Autodesk Fusion 360 part; units mm, degrees
(part 5 of 7)
  line L387 (58.5414, -43.6372) -> (58.5794, -43.7007)
  line L388 (58.5794, -43.7007) -> (58.6195, -43.7622)
  line L389 (58.6195, -43.7622) -> (58.6622, -43.8212)
  line L390 (58.6622, -43.8212) -> (58.7086, -43.8765)
  line L391 (58.7086, -43.8765) -> (59.0247, -44.1929)
  line L392 (59.0247, -44.1929) -> (58.8773, -44.3441)
  line L393 (58.8773, -44.3441) -> (58.734, -44.4991)
  line L394 (58.734, -44.4991) -> (58.5948, -44.6578)
  line L395 (58.5948, -44.6578) -> (58.4598, -44.8202)
  line L396 (58.4598, -44.8202) -> (58.1122, -44.5389)
  line L397 (58.1122, -44.5389) -> (58.0523, -44.4985)
  line L398 (58.0523, -44.4985) -> (57.9892, -44.4623)
  line L399 (57.9892, -44.4623) -> (57.9238, -44.4288)
  line L400 (57.9238, -44.4288) -> (57.8567, -44.3976)
  line L401 (57.8567, -44.3976) -> (57.788, -44.3685)
  line L402 (57.788, -44.3685) -> (57.7178, -44.3412)
  line L403 (57.7178, -44.3412) -> (57.6464, -44.3157)
  line L404 (57.6464, -44.3157) -> (57.5738, -44.2918)
  line L405 (57.5738, -44.2918) -> (57.5, -44.2695)
  line L406 (57.5, -44.2695) -> (57.4251, -44.2487)
  line L407 (57.4251, -44.2487) -> (57.3492, -44.2295)
  line L408 (57.3492, -44.2295) -> (57.2723, -44.2117)
  line L409 (57.2723, -44.2117) -> (57.188, -44.324)
  line L410 (57.188, -44.324) -> (57.1055, -44.4376)
  line L411 (57.1055, -44.4376) -> (57.0247, -44.5525)
  line L412 (57.0247, -44.5525) -> (57.0654, -44.6201)
  line L413 (57.0654, -44.6201) -> (57.1071, -44.6863)
  line L414 (57.1071, -44.6863) -> (57.15, -44.7511)
  line L415 (57.15, -44.7511) -> (57.194, -44.8144)
  line L416 (57.194, -44.8144) -> (57.2392, -44.8762)
  line L417 (57.2392, -44.8762) -> (57.2856, -44.9362)
  line L418 (57.2856, -44.9362) -> (57.3332, -44.9945)
  line L419 (57.3332, -44.9945) -> (57.3821, -45.0508)
  line L420 (57.3821, -45.0508) -> (57.4325, -45.105)
  line L421 (57.4325, -45.105) -> (57.4846, -45.1568)
  line L422 (57.4846, -45.1568) -> (57.5385, -45.2057)
  line L423 (57.5385, -45.2057) -> (57.5954, -45.2502)
  line L424 (57.5954, -45.2502) -> (57.9704, -45.4939)
  line L425 (57.9704, -45.4939) -> (57.8577, -45.6724)
  line L426 (57.8577, -45.6724) -> (57.7497, -45.8538)
  line L427 (57.7497, -45.8538) -> (57.6466, -46.038)
  line L428 (57.6466, -46.038) -> (57.5483, -46.2249)
  line L429 (57.5483, -46.2249) -> (57.1498, -46.022)
  line L430 (57.1498, -46.022) -> (57.0828, -45.995)
  line L431 (57.0828, -45.995) -> (57.0135, -45.9727)
  line L432 (57.0135, -45.9727) -> (56.9427, -45.9535)
  line L433 (56.9427, -45.9535) -> (56.8705, -45.937)
  line L434 (56.8705, -45.937) -> (56.7972, -45.9228)
  line L435 (56.7972, -45.9228) -> (56.723, -45.9107)
  line L436 (56.723, -45.9107) -> (56.6478, -45.9005)
  line L437 (56.6478, -45.9005) -> (56.5717, -45.8923)
  line L438 (56.5717, -45.8923) -> (56.4949, -45.8858)
  line L439 (56.4949, -45.8858) -> (56.4174, -45.8811)
  line L440 (56.4174, -45.8811) -> (56.3391, -45.878)
  line L441 (56.3391, -45.878) -> (56.2602, -45.8766)
  line L442 (56.2602, -45.8766) -> (56.2011, -46.004)
  line L443 (56.2011, -46.004) -> (56.144, -46.1323)
  line L444 (56.144, -46.1323) -> (56.0888, -46.2614)
  line L445 (56.0888, -46.2614) -> (56.1427, -46.3191)
  line L446 (56.1427, -46.3191) -> (56.1973, -46.3752)
  line L447 (56.1973, -46.3752) -> (56.2528, -46.4297)
  line L448 (56.2528, -46.4297) -> (56.309, -46.4825)
  line L449 (56.309, -46.4825) -> (56.366, -46.5334)
  line L450 (56.366, -46.5334) -> (56.4238, -46.5825)
  line L451 (56.4238, -46.5825) -> (56.4825, -46.6296)
  line L452 (56.4825, -46.6296) -> (56.5421, -46.6746)
  line L453 (56.5421, -46.6746) -> (56.6027, -46.7171)
  line L454 (56.6027, -46.7171) -> (56.6644, -46.757)
  line L455 (56.6644, -46.757) -> (56.7273, -46.7936)
  line L456 (56.7273, -46.7936) -> (56.7922, -46.8252)
  line L457 (56.7922, -46.8252) -> (57.2096, -46.9856)
  line L458 (57.2096, -46.9856) -> (57.1365, -47.1837)
  line L459 (57.1365, -47.1837) -> (57.0686, -47.3836)
  line L460 (57.0686, -47.3836) -> (57.006, -47.5852)
  line L461 (57.006, -47.5852) -> (56.9488, -47.7885)
  line L462 (56.9488, -47.7885) -> (56.5167, -47.6729)
  line L463 (56.5167, -47.6729) -> (56.4457, -47.6603)
  line L464 (56.4457, -47.6603) -> (56.3732, -47.6529)
  line L465 (56.3732, -47.6529) -> (56.2999, -47.6489)
  line L466 (56.2999, -47.6489) -> (56.2259, -47.6478)
  line L467 (56.2259, -47.6478) -> (56.1513, -47.6491)
  line L468 (56.1513, -47.6491) -> (56.0761, -47.6527)
  line L469 (56.0761, -47.6527) -> (56.0005, -47.6584)
  line L470 (56.0005, -47.6584) -> (55.9244, -47.6661)
  line L471 (55.9244, -47.6661) -> (55.8479, -47.6758)
  line L472 (55.8479, -47.6758) -> (55.771, -47.6873)
  line L473 (55.771, -47.6873) -> (55.6939, -47.7005)
  line L474 (55.6939, -47.7005) -> (55.6164, -47.7156)
  line L475 (55.6164, -47.7156) -> (55.5851, -47.8525)
  line L476 (55.5851, -47.8525) -> (55.5559, -47.9898)
  line L477 (55.5559, -47.9898) -> (55.5288, -48.1276)
  line L478 (55.5288, -48.1276) -> (55.5935, -48.1728)
  line L479 (55.5935, -48.1728) -> (55.6586, -48.2164)
  line L480 (55.6586, -48.2164) -> (55.7241, -48.2581)
  line L481 (55.7241, -48.2581) -> (55.79, -48.2981)
  line L482 (55.79, -48.2981) -> (55.8564, -48.3361)
  line L483 (55.8564, -48.3361) -> (55.9232, -48.3721)
  line L484 (55.9232, -48.3721) -> (55.9904, -48.4059)
  line L485 (55.9904, -48.4059) -> (56.058, -48.4375)
  line L486 (56.058, -48.4375) -> (56.1261, -48.4665)
  line L487 (56.1261, -48.4665) -> (56.1947, -48.4927)
  line L488 (56.1947, -48.4927) -> (56.2639, -48.5154)
  line L489 (56.2639, -48.5154) -> (56.3339, -48.5328)
  line L490 (56.3339, -48.5328) -> (56.7757, -48.603)
  line L491 (56.7757, -48.603) -> (56.7453, -48.8119)
  line L492 (56.7453, -48.8119) -> (56.7205, -49.0216)
  line L493 (56.7205, -49.0216) -> (56.7012, -49.2318)
  line L494 (56.7012, -49.2318) -> (56.6874, -49.4425)
  line L495 (56.6874, -49.4425) -> (56.2408, -49.4192)
  line L496 (56.2408, -49.4192) -> (56.1687, -49.4218)
  line L497 (56.1687, -49.4218) -> (56.0963, -49.4296)
  line L498 (56.0963, -49.4296) -> (56.0237, -49.4409)
  line L499 (56.0237, -49.4409) -> (55.9511, -49.4551)
  line L500 (55.9511, -49.4551) -> (55.8784, -49.472)
  line L501 (55.8784, -49.472) -> (55.8056, -49.4911)
  line L502 (55.8056, -49.4911) -> (55.7328, -49.5124)
  line L503 (55.7328, -49.5124) -> (55.66, -49.5358)
  line L504 (55.66, -49.5358) -> (55.5871, -49.5611)
  line L505 (55.5871, -49.5611) -> (55.5144, -49.5884)
  line L506 (55.5144, -49.5884) -> (55.4416, -49.6174)
  line L507 (55.4416, -49.6174) -> (55.369, -49.6482)
  line L508 (55.369, -49.6482) -> (55.3669, -49.7886)
  line L509 (55.3669, -49.7886) -> (55.3669, -49.929)
  line L510 (55.3669, -49.929) -> (55.369, -50.0695)
  line L511 (55.369, -50.0695) -> (55.4416, -50.1003)
  line L512 (55.4416, -50.1003) -> (55.5144, -50.1293)
  line L513 (55.5144, -50.1293) -> (55.5871, -50.1565)
  line L514 (55.5871, -50.1565) -> (55.66, -50.1819)
  line L515 (55.66, -50.1819) -> (55.7328, -50.2052)
  line L516 (55.7328, -50.2052) -> (55.8056, -50.2266)
  line L517 (55.8056, -50.2266) -> (55.8784, -50.2457)
  line L518 (55.8784, -50.2457) -> (55.9511, -50.2625)
  line L519 (55.9511, -50.2625) -> (56.0237, -50.2768)
  line L520 (56.0237, -50.2768) -> (56.0963, -50.2881)
  line L521 (56.0963, -50.2881) -> (56.1687, -50.2959)
  line L522 (56.1687, -50.2959) -> (56.2408, -50.2984)
  line L523 (56.2408, -50.2984) -> (56.6874, -50.2752)
  line L524 (56.6874, -50.2752) -> (56.7012, -50.4859)
  line L525 (56.7012, -50.4859) -> (56.7205, -50.6961)
  line L526 (56.7205, -50.6961) -> (56.7453, -50.9058)
  line L527 (56.7453, -50.9058) -> (56.7757, -51.1147)
  line L528 (56.7757, -51.1147) -> (56.3339, -51.1848)
  line L529 (56.3339, -51.1848) -> (56.2639, -51.2023)
  line L530 (56.2639, -51.2023) -> (56.1947, -51.225)
  line L531 (56.1947, -51.225) -> (56.1261, -51.2511)
  line L532 (56.1261, -51.2511) -> (56.058, -51.2802)
  line L533 (56.058, -51.2802) -> (55.9904, -51.3117)
  line L534 (55.9904, -51.3117) -> (55.9232, -51.3456)
  line L535 (55.9232, -51.3456) -> (55.8564, -51.3816)
  line L536 (55.8564, -51.3816) -> (55.79, -51.4196)
  line L537 (55.79, -51.4196) -> (55.7241, -51.4595)
  line L538 (55.7241, -51.4595) -> (55.6586, -51.5013)
  line L539 (55.6586, -51.5013) -> (55.5935, -51.5448)
  line L540 (55.5935, -51.5448) -> (55.5288, -51.59)
  line L541 (55.5288, -51.59) -> (55.5559, -51.7278)
  line L542 (55.5559, -51.7278) -> (55.5851, -51.8652)
  line L543 (55.5851, -51.8652) -> (55.6164, -52.0021)
  line L544 (55.6164, -52.0021) -> (55.6939, -52.0171)
  line L545 (55.6939, -52.0171) -> (55.771, -52.0304)
  line L546 (55.771, -52.0304) -> (55.8479, -52.0419)
  line L547 (55.8479, -52.0419) -> (55.9244, -52.0515)
  line L548 (55.9244, -52.0515) -> (56.0005, -52.0593)
  line L549 (56.0005, -52.0593) -> (56.0761, -52.065)
  line L550 (56.0761, -52.065) -> (56.1513, -52.0686)
  line L551 (56.1513, -52.0686) -> (56.2259, -52.0699)
  line L552 (56.2259, -52.0699) -> (56.2999, -52.0687)
  line L553 (56.2999, -52.0687) -> (56.3732, -52.0647)
  line L554 (56.3732, -52.0647) -> (56.4457, -52.0573)
  line L555 (56.4457, -52.0573) -> (56.5167, -52.0448)
  line L556 (56.5167, -52.0448) -> (56.9488, -51.9292)
  line L557 (56.9488, -51.9292) -> (57.006, -52.1324)
  line L558 (57.006, -52.1324) -> (57.0686, -52.3341)
  line L559 (57.0686, -52.3341) -> (57.1365, -52.534)
  line L560 (57.1365, -52.534) -> (57.2096, -52.732)
  line L561 (57.2096, -52.732) -> (56.7922, -52.8925)
  line L562 (56.7922, -52.8925) -> (56.7273, -52.9241)
  line L563 (56.7273, -52.9241) -> (56.6644, -52.9607)
  line L564 (56.6644, -52.9607) -> (56.6027, -53.0005)
  line L565 (56.6027, -53.0005) -> (56.5421, -53.0431)
  line L566 (56.5421, -53.0431) -> (56.4825, -53.088)
  line L567 (56.4825, -53.088) -> (56.4238, -53.1351)
  line L568 (56.4238, -53.1351) -> (56.366, -53.1842)
  line L569 (56.366, -53.1842) -> (56.309, -53.2352)
  line L570 (56.309, -53.2352) -> (56.2528, -53.288)
  line L571 (56.2528, -53.288) -> (56.1973, -53.3424)
  line L572 (56.1973, -53.3424) -> (56.1427, -53.3985)
  line L573 (56.1427, -53.3985) -> (56.0888, -53.4562)
  line L574 (56.0888, -53.4562) -> (56.144, -53.5854)
  line L575 (56.144, -53.5854) -> (56.2011, -53.7137)
  line L576 (56.2011, -53.7137) -> (56.2602, -53.8411)
  line L577 (56.2602, -53.8411) -> (56.3391, -53.8396)
  line L578 (56.3391, -53.8396) -> (56.4174, -53.8366)
  line L579 (56.4174, -53.8366) -> (56.4949, -53.8319)
  line L580 (56.4949, -53.8319) -> (56.5717, -53.8254)
  line L581 (56.5717, -53.8254) -> (56.6478, -53.8171)
  line L582 (56.6478, -53.8171) -> (56.723, -53.807)
  line L583 (56.723, -53.807) -> (56.7972, -53.7949)
  line L584 (56.7972, -53.7949) -> (56.8705, -53.7807)
  line L585 (56.8705, -53.7807) -> (56.9427, -53.7641)
  line L586 (56.9427, -53.7641) -> (57.0135, -53.745)
  line L587 (57.0135, -53.745) -> (57.0828, -53.7227)
  line L588 (57.0828, -53.7227) -> (57.1498, -53.6956)
  line L589 (57.1498, -53.6956) -> (57.5483, -53.4927)
  line L590 (57.5483, -53.4927) -> (57.6466, -53.6796)
  line L591 (57.6466, -53.6796) -> (57.7497, -53.8638)
  line L592 (57.7497, -53.8638) -> (57.8577, -54.0453)
  line L593 (57.8577, -54.0453) -> (57.9704, -54.2238)
  line L594 (57.9704, -54.2238) -> (57.5954, -54.4675)
  line L595 (57.5954, -54.4675) -> (57.5385, -54.5119)
  line L596 (57.5385, -54.5119) -> (57.4846, -54.5608)
  line L597 (57.4846, -54.5608) -> (57.4325, -54.6126)
  line L598 (57.4325, -54.6126) -> (57.3821, -54.6668)
  line L599 (57.3821, -54.6668) -> (57.3332, -54.7232)
  line L600 (57.3332, -54.7232) -> (57.2856, -54.7815)
  line L601 (57.2856, -54.7815) -> (57.2392, -54.8415)
  line L602 (57.2392, -54.8415) -> (57.194, -54.9032)
  line L603 (57.194, -54.9032) -> (57.15, -54.9665)
  line L604 (57.15, -54.9665) -> (57.1071, -55.0313)
  line L605 (57.1071, -55.0313) -> (57.0654, -55.0976)
  line L606 (57.0654, -55.0976) -> (57.0247, -55.1652)
  line L607 (57.0247, -55.1652) -> (57.1055, -55.28)
  line L608 (57.1055, -55.28) -> (57.188, -55.3936)
  line L609 (57.188, -55.3936) -> (57.2723, -55.506)
  line L610 (57.2723, -55.506) -> (57.3492, -55.4882)
  line L611 (57.3492, -55.4882) -> (57.4251, -55.4689)
  line L612 (57.4251, -55.4689) -> (57.5, -55.4482)
  line L613 (57.5, -55.4482) -> (57.5738, -55.4259)
  line L614 (57.5738, -55.4259) -> (57.6464, -55.402)
  line L615 (57.6464, -55.402) -> (57.7178, -55.3765)
  line L616 (57.7178, -55.3765) -> (57.788, -55.3492)
  line L617 (57.788, -55.3492) -> (57.8567, -55.32)
  line L618 (57.8567, -55.32) -> (57.9238, -55.2888)
  line L619 (57.9238, -55.2888) -> (57.9892, -55.2554)
  line L620 (57.9892, -55.2554) -> (58.0523, -55.2191)
  line L621 (58.0523, -55.2191) -> (58.1122, -55.1788)
  line L622 (58.1122, -55.1788) -> (58.4598, -54.8975)
  line L623 (58.4598, -54.8975) -> (58.5948, -55.0598)
  line L624 (58.5948, -55.0598) -> (58.734, -55.2186)
  line L625 (58.734, -55.2186) -> (58.8773, -55.3736)
  line L626 (58.8773, -55.3736) -> (59.0247, -55.5248)
  line L627 (59.0247, -55.5248) -> (58.7086, -55.8411)
  line L628 (58.7086, -55.8411) -> (58.6622, -55.8964)
  line L629 (58.6622, -55.8964) -> (58.6195, -55.9554)
  line L630 (58.6195, -55.9554) -> (58.5794, -56.0169)
  line L631 (58.5794, -56.0169) -> (58.5414, -56.0805)
  line L632 (58.5414, -56.0805) -> (58.5052, -56.1457)
  line L633 (58.5052, -56.1457) -> (58.4708, -56.2126)
  line L634 (58.4708, -56.2126) -> (58.4379, -56.281)
  line L635 (58.4379, -56.281) -> (58.4065, -56.3508)
  line L636 (58.4065, -56.3508) -> (58.3767, -56.4218)
  line L637 (58.3767, -56.4218) -> (58.3482, -56.4941)
  line L638 (58.3482, -56.4941) -> (58.3211, -56.5676)
  line L639 (58.3211, -56.5676) -> (58.2954, -56.6422)
  line L640 (58.2954, -56.6422) -> (58.3983, -56.7378)
  line L641 (58.3983, -56.7378) -> (58.5026, -56.8317)
  line L642 (58.5026, -56.8317) -> (58.6084, -56.9241)
  line L643 (58.6084, -56.9241) -> (58.6799, -56.8907)
  line L644 (58.6799, -56.8907) -> (58.7502, -56.8561)
  line L645 (58.7502, -56.8561) -> (58.8191, -56.8202)
  line L646 (58.8191, -56.8202) -> (58.8866, -56.7831)
  line L647 (58.8866, -56.7831) -> (58.9527, -56.7446)
  line L648 (58.9527, -56.7446) -> (59.0173, -56.7048)
  line L649 (59.0173, -56.7048) -> (59.0802, -56.6635)
  line L650 (59.0802, -56.6635) -> (59.1414, -56.6207)
  line L651 (59.1414, -56.6207) -> (59.2006, -56.5762)
  line L652 (59.2006, -56.5762) -> (59.2575, -56.5299)
  line L653 (59.2575, -56.5299) -> (59.3118, -56.4813)
  line L654 (59.3118, -56.4813) -> (59.3619, -56.4294)
  line L655 (59.3619, -56.4294) -> (59.6435, -56.082)
  line L656 (59.6435, -56.082) -> (59.8093, -56.2127)
  line L657 (59.8093, -56.2127) -> (59.9784, -56.3391)
  line L658 (59.9784, -56.3391) -> (60.1509, -56.4609)
  line L659 (60.1509, -56.4609) -> (60.3264, -56.5781)
  line L660 (60.3264, -56.5781) -> (60.083, -56.9533)
  line L661 (60.083, -56.9533) -> (60.0491, -57.017)
  line L662 (60.0491, -57.017) -> (60.0197, -57.0836)
  line L663 (60.0197, -57.0836) -> (59.9932, -57.1521)
  line L664 (59.9932, -57.1521) -> (59.9692, -57.2222)
  line L665 (59.9692, -57.2222) -> (59.9474, -57.2935)
  line L666 (59.9474, -57.2935) -> (59.9276, -57.3661)
  line L667 (59.9276, -57.3661) -> (59.9097, -57.4399)
  line L668 (59.9097, -57.4399) -> (59.8935, -57.5146)
  line L669 (59.8935, -57.5146) -> (59.8791, -57.5903)
  line L670 (59.8791, -57.5903) -> (59.8663, -57.667)
  line L671 (59.8663, -57.667) -> (59.855, -57.7445)
  line L672 (59.855, -57.7445) -> (59.8454, -57.8228)
  line L673 (59.8454, -57.8228) -> (59.9659, -57.8949)
  line L674 (59.9659, -57.8949) -> (60.0875, -57.9651)
  line L675 (60.0875, -57.9651) -> (60.2102, -58.0334)
  line L676 (60.2102, -58.0334) -> (60.2732, -57.9859)
  line L677 (60.2732, -57.9859) -> (60.3347, -57.9374)
  line L678 (60.3347, -57.9374) -> (60.3947, -57.888)
  line L679 (60.3947, -57.888) -> (60.453, -57.8376)
  line L680 (60.453, -57.8376) -> (60.5097, -57.7863)
  line L681 (60.5097, -57.7863) -> (60.5645, -57.7339)
  line L682 (60.5645, -57.7339) -> (60.6175, -57.6804)
  line L683 (60.6175, -57.6804) -> (60.6684, -57.6258)
  line L684 (60.6684, -57.6258) -> (60.7171, -57.57)
  line L685 (60.7171, -57.57) -> (60.7632, -57.5129)
  line L686 (60.7632, -57.5129) -> (60.8061, -57.4541)
  line L687 (60.8061, -57.4541) -> (60.8444, -57.3929)
  line L688 (60.8444, -57.3929) -> (61.0476, -56.9945)
  line L689 (61.0476, -56.9945) -> (61.2369, -57.0879)
  line L690 (61.2369, -57.0879) -> (61.4286, -57.1763)
  line L691 (61.4286, -57.1763) -> (61.6226, -57.2597)
  line L692 (61.6226, -57.2597) -> (61.8187, -57.3378)
  line L693 (61.8187, -57.3378) -> (61.6586, -57.7554)
  line L694 (61.6586, -57.7554) -> (61.6387, -57.8248)
  line L695 (61.6387, -57.8248) -> (61.6238, -57.8961)
  line L696 (61.6238, -57.8961) -> (61.6121, -57.9685)
  line L697 (61.6121, -57.9685) -> (61.6032, -58.042)
  line L698 (61.6032, -58.042) -> (61.5968, -58.1164)
  line L699 (61.5968, -58.1164) -> (61.5925, -58.1915)
  line L700 (61.5925, -58.1915) -> (61.5903, -58.2674)
  line L701 (61.5903, -58.2674) -> (61.59, -58.3438)
  line L702 (61.59, -58.3438) -> (61.5916, -58.4209)
  line L703 (61.5916, -58.4209) -> (61.595, -58.4986)
  line L704 (61.595, -58.4986) -> (61.6001, -58.5767)
  line L705 (61.6001, -58.5767) -> (61.607, -58.6553)
  line L706 (61.607, -58.6553) -> (61.7399, -58.7007)
  line L707 (61.7399, -58.7007) -> (61.8734, -58.7441)
  line L708 (61.8734, -58.7441) -> (62.0076, -58.7855)
  line L709 (62.0076, -58.7855) -> (62.0593, -58.7259)
  line L710 (62.0593, -58.7259) -> (62.1094, -58.6657)
  line L711 (62.1094, -58.6657) -> (62.1578, -58.6049)
  line L712 (62.1578, -58.6049) -> (62.2044, -58.5435)
  line L713 (62.2044, -58.5435) -> (62.2492, -58.4815)
  line L714 (62.2492, -58.4815) -> (62.2919, -58.4188)
  line L715 (62.2919, -58.4188) -> (62.3326, -58.3555)
  line L716 (62.3326, -58.3555) -> (62.3711, -58.2915)
  line L717 (62.3711, -58.2915) -> (62.4071, -58.2268)
  line L718 (62.4071, -58.2268) -> (62.4403, -58.1613)
  line L719 (62.4403, -58.1613) -> (62.4701, -58.0949)
  line L720 (62.4701, -58.0949) -> (62.4948, -58.0271)
  line L721 (62.4948, -58.0271) -> (62.6107, -57.5952)
  line L722 (62.6107, -57.5952) -> (62.8153, -57.6472)
  line L723 (62.8153, -57.6472) -> (63.0212, -57.6938)
  line L724 (63.0212, -57.6938) -> (63.2283, -57.735)
  line L725 (63.2283, -57.735) -> (63.4364, -57.7707)
  line L726 (63.4364, -57.7707) -> (63.3666, -58.2124)
  line L727 (63.3666, -58.2124) -> (63.3615, -58.2844)
  line L728 (63.3615, -58.2844) -> (63.3617, -58.3572)
  line L729 (63.3617, -58.3572) -> (63.3654, -58.4305)
  line L730 (63.3654, -58.4305) -> (63.372, -58.5043)
  line L731 (63.372, -58.5043) -> (63.3811, -58.5784)
  line L732 (63.3811, -58.5784) -> (63.3926, -58.6527)
  line L733 (63.3926, -58.6527) -> (63.4062, -58.7274)
  line L734 (63.4062, -58.7274) -> (63.4218, -58.8022)
  line L735 (63.4218, -58.8022) -> (63.4394, -58.8773)
  line L736 (63.4394, -58.8773) -> (63.4588, -58.9525)
  line L737 (63.4588, -58.9525) -> (63.4801, -59.0279)
  line L738 (63.4801, -59.0279) -> (63.5032, -59.1034)
  line L739 (63.5032, -59.1034) -> (63.6426, -59.1202)
  line L740 (63.6426, -59.1202) -> (63.7822, -59.1349)
  line L741 (63.7822, -59.1349) -> (63.9221, -59.1474)
  line L742 (63.9221, -59.1474) -> (63.9603, -59.0784)
  line L743 (63.9603, -59.0784) -> (63.9968, -59.0091)
  line L744 (63.9968, -59.0091) -> (64.0315, -58.9395)
  line L745 (64.0315, -58.9395) -> (64.0643, -58.8698)
  line L746 (64.0643, -58.8698) -> (64.0952, -58.7998)
  line L747 (64.0952, -58.7998) -> (64.124, -58.7296)
  line L748 (64.124, -58.7296) -> (64.1506, -58.6592)
  line L749 (64.1506, -58.6592) -> (64.175, -58.5887)
  line L750 (64.175, -58.5887) -> (64.1967, -58.5179)
  line L751 (64.1967, -58.5179) -> (64.2156, -58.447)
  line L752 (64.2156, -58.447) -> (64.2309, -58.3758)
  line L753 (64.2309, -58.3758) -> (64.241, -58.3043)
  line L754 (64.241, -58.3043) -> (64.2645, -57.8577)
  line L755 (64.2645, -57.8577) -> (64.4755, -57.866)
  line L756 (64.4755, -57.866) -> (64.6866, -57.8688)
  line L757 (64.6866, -57.8688) -> (64.8977, -57.866)
  line L758 (64.8977, -57.866) -> (65.1087, -57.8577)
  line L759 (65.1087, -57.8577) -> (65.1322, -58.3043)
  line L760 (65.1322, -58.3043) -> (65.1423, -58.3758)
  line L761 (65.1423, -58.3758) -> (65.1576, -58.447)
  line L762 (65.1576, -58.447) -> (65.1765, -58.5179)
  line L763 (65.1765, -58.5179) -> (65.1982, -58.5887)
  line L764 (65.1982, -58.5887) -> (65.2225, -58.6592)
  line L765 (65.2225, -58.6592) -> (65.2492, -58.7296)
  line L766 (65.2492, -58.7296) -> (65.278, -58.7998)
  line L767 (65.278, -58.7998) -> (65.3089, -58.8698)
  line L768 (65.3089, -58.8698) -> (65.3417, -58.9395)
  line L769 (65.3417, -58.9395) -> (65.3764, -59.0091)
  line L770 (65.3764, -59.0091) -> (65.4128, -59.0784)
  line L771 (65.4128, -59.0784) -> (65.4511, -59.1474)
  line L772 (65.4511, -59.1474) -> (65.5909, -59.1349)
  line L773 (65.5909, -59.1349) -> (65.7306, -59.1202)
  line L774 (65.7306, -59.1202) -> (65.87, -59.1034)
  line L775 (65.87, -59.1034) -> (65.8931, -59.0279)
  line L776 (65.8931, -59.0279) -> (65.9143, -58.9525)
  line L777 (65.9143, -58.9525) -> (65.9338, -58.8773)
  line L778 (65.9338, -58.8773) -> (65.9514, -58.8022)
  line L779 (65.9514, -58.8022) -> (65.967, -58.7274)
  line L780 (65.967, -58.7274) -> (65.9806, -58.6527)
  line L781 (65.9806, -58.6527) -> (65.9921, -58.5784)
  line L782 (65.9921, -58.5784) -> (66.0012, -58.5043)
  line L783 (66.0012, -58.5043) -> (66.0077, -58.4305)
  line L784 (66.0077, -58.4305) -> (66.0114, -58.3572)
  line L785 (66.0114, -58.3572) -> (66.0116, -58.2844)
  line L786 (66.0116, -58.2844) -> (66.0066, -58.2124)
  line L787 (66.0066, -58.2124) -> (65.9368, -57.7707)
  line L788 (65.9368, -57.7707) -> (66.1449, -57.735)
  line L789 (66.1449, -57.735) -> (66.352, -57.6938)
  line L790 (66.352, -57.6938) -> (66.5579, -57.6472)
  line L791 (66.5579, -57.6472) -> (66.7625, -57.5952)
  line L792 (66.7625, -57.5952) -> (66.8784, -58.0271)
  line L793 (66.8784, -58.0271) -> (66.9031, -58.0949)
  line L794 (66.9031, -58.0949) -> (66.9329, -58.1613)
  line L795 (66.9329, -58.1613) -> (66.9661, -58.2268)
  line L796 (66.9661, -58.2268) -> (67.0021, -58.2915)
  line L797 (67.0021, -58.2915) -> (67.0405, -58.3555)
  line L798 (67.0405, -58.3555) -> (67.0812, -58.4188)
  line L799 (67.0812, -58.4188) -> (67.124, -58.4815)
  line L800 (67.124, -58.4815) -> (67.1688, -58.5435)
  line L801 (67.1688, -58.5435) -> (67.2154, -58.6049)
  line L802 (67.2154, -58.6049) -> (67.2637, -58.6657)
  line L803 (67.2637, -58.6657) -> (67.3138, -58.7259)
  line L804 (67.3138, -58.7259) -> (67.3656, -58.7855)
  line L805 (67.3656, -58.7855) -> (67.4998, -58.7441)
  line L806 (67.4998, -58.7441) -> (67.6333, -58.7007)
  line L807 (67.6333, -58.7007) -> (67.7662, -58.6553)
  line L808 (67.7662, -58.6553) -> (67.773, -58.5767)
  line L809 (67.773, -58.5767) -> (67.7782, -58.4986)
  line L810 (67.7782, -58.4986) -> (67.7816, -58.4209)
  line L811 (67.7816, -58.4209) -> (67.7832, -58.3438)
  line L812 (67.7832, -58.3438) -> (67.7829, -58.2674)
  line L813 (67.7829, -58.2674) -> (67.7807, -58.1915)
  line L814 (67.7807, -58.1915) -> (67.7764, -58.1164)
  line L815 (67.7764, -58.1164) -> (67.7699, -58.042)
  line L816 (67.7699, -58.042) -> (67.761, -57.9685)
  line L817 (67.761, -57.9685) -> (67.7494, -57.8961)
  line L818 (67.7494, -57.8961) -> (67.7344, -57.8248)
  line L819 (67.7344, -57.8248) -> (67.7146, -57.7554)
  line L820 (67.7146, -57.7554) -> (67.5544, -57.3378)
  line L821 (67.5544, -57.3378) -> (67.7506, -57.2597)
  line L822 (67.7506, -57.2597) -> (67.9445, -57.1763)
  line L823 (67.9445, -57.1763) -> (68.1363, -57.0879)
  line L824 (68.1363, -57.0879) -> (68.3256, -56.9945)
  line L825 (68.3256, -56.9945) -> (68.5288, -57.3929)
  line L826 (68.5288, -57.3929) -> (68.567, -57.4541)
  line L827 (68.567, -57.4541) -> (68.61, -57.5129)
  line L828 (68.61, -57.5129) -> (68.6561, -57.57)
  line L829 (68.6561, -57.57) -> (68.7047, -57.6258)
  line L830 (68.7047, -57.6258) -> (68.7557, -57.6804)
  line L831 (68.7557, -57.6804) -> (68.8086, -57.7339)
  line L832 (68.8086, -57.7339) -> (68.8635, -57.7863)
  line L833 (68.8635, -57.7863) -> (68.9202, -57.8376)
  line L834 (68.9202, -57.8376) -> (68.9785, -57.888)
  line L835 (68.9785, -57.888) -> (69.0385, -57.9374)
  line L836 (69.0385, -57.9374) -> (69.1, -57.9859)
  line L837 (69.1, -57.9859) -> (69.163, -58.0334)
  line L838 (69.163, -58.0334) -> (69.2856, -57.9651)
  line L839 (69.2856, -57.9651) -> (69.4073, -57.8949)
  line L840 (69.4073, -57.8949) -> (69.5278, -57.8228)
  line L841 (69.5278, -57.8228) -> (69.5181, -57.7445)
  line L842 (69.5181, -57.7445) -> (69.5069, -57.667)
  line L843 (69.5069, -57.667) -> (69.4941, -57.5903)
  line L844 (69.4941, -57.5903) -> (69.4796, -57.5146)
  line L845 (69.4796, -57.5146) -> (69.4635, -57.4399)
  line L846 (69.4635, -57.4399) -> (69.4456, -57.3661)
  line L847 (69.4456, -57.3661) -> (69.4257, -57.2935)
  line L848 (69.4257, -57.2935) -> (69.4039, -57.2222)
  line L849 (69.4039, -57.2222) -> (69.3799, -57.1521)
  line L850 (69.3799, -57.1521) -> (69.3535, -57.0836)
  line L851 (69.3535, -57.0836) -> (69.3241, -57.017)
  line L852 (69.3241, -57.017) -> (69.2902, -56.9533)
  line L853 (69.2902, -56.9533) -> (69.0467, -56.5781)
  line L854 (69.0467, -56.5781) -> (69.2223, -56.4609)
  line L855 (69.2223, -56.4609) -> (69.3947, -56.3391)
  line L856 (69.3947, -56.3391) -> (69.5639, -56.2127)
  line L857 (69.5639, -56.2127) -> (69.7297, -56.082)
  line L858 (69.7297, -56.082) -> (70.0112, -56.4294)
  line L859 (70.0112, -56.4294) -> (70.0614, -56.4813)
  line L860 (70.0614, -56.4813) -> (70.1156, -56.5299)
  line L861 (70.1156, -56.5299) -> (70.1726, -56.5762)
  line L862 (70.1726, -56.5762) -> (70.2318, -56.6207)
  line L863 (70.2318, -56.6207) -> (70.2929, -56.6635)
  line L864 (70.2929, -56.6635) -> (70.3559, -56.7048)
  line L865 (70.3559, -56.7048) -> (70.4204, -56.7446)
  line L866 (70.4204, -56.7446) -> (70.4865, -56.7831)
  line L867 (70.4865, -56.7831) -> (70.5541, -56.8202)
  line L868 (70.5541, -56.8202) -> (70.623, -56.8561)
  line L869 (70.623, -56.8561) -> (70.6933, -56.8907)
  line L870 (70.6933, -56.8907) -> (70.7648, -56.9241)
  line L871 (70.7648, -56.9241) -> (70.8705, -56.8317)
  line L872 (70.8705, -56.8317) -> (70.9749, -56.7378)
  line L873 (70.9749, -56.7378) -> (71.0778, -56.6422)
  line L874 (71.0778, -56.6422) -> (71.0521, -56.5676)
  line L875 (71.0521, -56.5676) -> (71.025, -56.4941)
  line L876 (71.025, -56.4941) -> (70.9965, -56.4218)
  line L877 (70.9965, -56.4218) -> (70.9666, -56.3508)
  line L878 (70.9666, -56.3508) -> (70.9353, -56.281)
  line L879 (70.9353, -56.281) -> (70.9024, -56.2126)
  line L880 (70.9024, -56.2126) -> (70.8679, -56.1457)
  line L881 (70.8679, -56.1457) -> (70.8318, -56.0805)
  line L882 (70.8318, -56.0805) -> (70.7937, -56.0169)
  line L883 (70.7937, -56.0169) -> (70.7536, -55.9554)
  line L884 (70.7536, -55.9554) -> (70.711, -55.8964)
  line L885 (70.711, -55.8964) -> (70.6646, -55.8411)
  line L886 (70.6646, -55.8411) -> (70.3485, -55.5248)
  line L887 (70.3485, -55.5248) -> (70.4959, -55.3736)
  line L888 (70.4959, -55.3736) -> (70.6392, -55.2186)
  line L889 (70.6392, -55.2186) -> (70.7784, -55.0598)
  line L890 (70.7784, -55.0598) -> (70.9133, -54.8975)
  line L891 (70.9133, -54.8975) -> (71.261, -55.1788)
  line L892 (71.261, -55.1788) -> (71.3208, -55.2191)
  line L893 (71.3208, -55.2191) -> (71.384, -55.2554)
  line L894 (71.384, -55.2554) -> (71.4493, -55.2888)
  line L895 (71.4493, -55.2888) -> (71.5165, -55.32)
  line L896 (71.5165, -55.32) -> (71.5852, -55.3492)
  line L897 (71.5852, -55.3492) -> (71.6553, -55.3765)
  line L898 (71.6553, -55.3765) -> (71.7268, -55.402)
  line L899 (71.7268, -55.402) -> (71.7994, -55.4259)
  line L900 (71.7994, -55.4259) -> (71.8732, -55.4482)
  line L901 (71.8732, -55.4482) -> (71.9481, -55.4689)
  line L902 (71.9481, -55.4689) -> (72.024, -55.4882)
  line L903 (72.024, -55.4882) -> (72.1009, -55.506)
  line L904 (72.1009, -55.506) -> (72.1851, -55.3936)
  line L905 (72.1851, -55.3936) -> (72.2677, -55.28)
  line L906 (72.2677, -55.28) -> (72.3485, -55.1652)
  line L907 (72.3485, -55.1652) -> (72.3078, -55.0976)
  line L908 (72.3078, -55.0976) -> (72.266, -55.0313)
  line L909 (72.266, -55.0313) -> (72.2232, -54.9665)
  line L910 (72.2232, -54.9665) -> (72.1792, -54.9032)
  line L911 (72.1792, -54.9032) -> (72.134, -54.8415)
  line L912 (72.134, -54.8415) -> (72.0876, -54.7815)
  line L913 (72.0876, -54.7815) -> (72.04, -54.7232)
  line L914 (72.04, -54.7232) -> (71.991, -54.6668)
  line L915 (71.991, -54.6668) -> (71.9406, -54.6126)
  line L916 (71.9406, -54.6126) -> (71.8886, -54.5608)
  line L917 (71.8886, -54.5608) -> (71.8346, -54.5119)
  line L918 (71.8346, -54.5119) -> (71.7778, -54.4675)
  line L919 (71.7778, -54.4675) -> (71.4028, -54.2238)
  line L920 (71.4028, -54.2238) -> (71.5155, -54.0453)
  line L921 (71.5155, -54.0453) -> (71.6234, -53.8638)
  line L922 (71.6234, -53.8638) -> (71.7266, -53.6796)
  line L923 (71.7266, -53.6796) -> (71.8248, -53.4927)
  line L924 (71.8248, -53.4927) -> (72.2234, -53.6956)
  line L925 (72.2234, -53.6956) -> (72.2903, -53.7227)
  line L926 (72.2903, -53.7227) -> (72.3596, -53.745)
  line L927 (72.3596, -53.745) -> (72.4305, -53.7641)
  line L928 (72.4305, -53.7641) -> (72.5027, -53.7807)
  line L929 (72.5027, -53.7807) -> (72.5759, -53.7949)
  line L930 (72.5759, -53.7949) -> (72.6502, -53.807)
  line L931 (72.6502, -53.807) -> (72.7254, -53.8171)
  line L932 (72.7254, -53.8171) -> (72.8014, -53.8254)
  line L933 (72.8014, -53.8254) -> (72.8783, -53.8319)
  line L934 (72.8783, -53.8319) -> (72.9558, -53.8366)
  line L935 (72.9558, -53.8366) -> (73.0341, -53.8396)
  line L936 (73.0341, -53.8396) -> (73.113, -53.8411)
  line L937 (73.113, -53.8411) -> (73.172, -53.7137)
  line L938 (73.172, -53.7137) -> (73.2291, -53.5854)
  line L939 (73.2291, -53.5854) -> (73.2843, -53.4562)
  line L940 (73.2843, -53.4562) -> (73.2305, -53.3985)
  line L941 (73.2305, -53.3985) -> (73.1758, -53.3424)
  line L942 (73.1758, -53.3424) -> (73.1204, -53.288)
  line L943 (73.1204, -53.288) -> (73.0642, -53.2352)
  line L944 (73.0642, -53.2352) -> (73.0072, -53.1842)
  line L945 (73.0072, -53.1842) -> (72.9494, -53.1351)
  line L946 (72.9494, -53.1351) -> (72.8907, -53.088)
  line L947 (72.8907, -53.088) -> (72.8311, -53.0431)
  line L948 (72.8311, -53.0431) -> (72.7705, -53.0005)
  line L949 (72.7705, -53.0005) -> (72.7088, -52.9607)
  line L950 (72.7088, -52.9607) -> (72.6459, -52.9241)
  line L951 (72.6459, -52.9241) -> (72.581, -52.8925)
  line L952 (72.581, -52.8925) -> (72.1635, -52.732)
  line L953 (72.1635, -52.732) -> (72.2367, -52.534)
  line L954 (72.2367, -52.534) -> (72.3045, -52.3341)
  line L955 (72.3045, -52.3341) -> (72.3671, -52.1324)
  line L956 (72.3671, -52.1324) -> (72.4244, -51.9292)
  line L957 (72.4244, -51.9292) -> (72.8564, -52.0448)
  line L958 (72.8564, -52.0448) -> (72.9275, -52.0573)
  line L959 (72.9275, -52.0573) -> (72.9999, -52.0647)
  line L960 (72.9999, -52.0647) -> (73.0732, -52.0687)
  line L961 (73.0732, -52.0687) -> (73.1473, -52.0699)
  line L962 (73.1473, -52.0699) -> (73.2219, -52.0686)
  line L963 (73.2219, -52.0686) -> (73.2971, -52.065)
  line L964 (73.2971, -52.065) -> (73.3727, -52.0593)
  line L965 (73.3727, -52.0593) -> (73.4488, -52.0515)
  line L966 (73.4488, -52.0515) -> (73.5253, -52.0419)
  line L967 (73.5253, -52.0419) -> (73.6021, -52.0304)
  line L968 (73.6021, -52.0304) -> (73.6793, -52.0171)
  line L969 (73.6793, -52.0171) -> (73.7568, -52.0021)
  line L970 (73.7568, -52.0021) -> (73.7881, -51.8652)
  line L971 (73.7881, -51.8652) -> (73.8173, -51.7278)
  line L972 (73.8173, -51.7278) -> (73.8444, -51.59)
  line L973 (73.8444, -51.59) -> (73.7797, -51.5448)
  line L974 (73.7797, -51.5448) -> (73.7146, -51.5013)
  line L975 (73.7146, -51.5013) -> (73.6491, -51.4595)
  line L976 (73.6491, -51.4595) -> (73.5831, -51.4196)
  line L977 (73.5831, -51.4196) -> (73.5168, -51.3816)
  line L978 (73.5168, -51.3816) -> (73.45, -51.3456)
  line L979 (73.45, -51.3456) -> (73.3828, -51.3117)
  line L980 (73.3828, -51.3117) -> (73.3151, -51.2802)
  line L981 (73.3151, -51.2802) -> (73.247, -51.2511)
  line L982 (73.247, -51.2511) -> (73.1784, -51.225)
  line L983 (73.1784, -51.225) -> (73.1092, -51.2023)
  line L984 (73.1092, -51.2023) -> (73.0392, -51.1848)
  line L985 (73.0392, -51.1848) -> (72.5975, -51.1147)
  line L986 (72.5975, -51.1147) -> (72.6279, -50.9058)
  line L987 (72.6279, -50.9058) -> (72.6527, -50.6961)
  line L988 (72.6527, -50.6961) -> (72.672, -50.4859)
  line L989 (72.672, -50.4859) -> (72.6858, -50.2752)
  circle A0 centre (64.6866, -49.8588) radius 1.5
extrude "Extrude1'''" add sketch "Sketch1 (4)" along normal blind 2 separate body makes body 8 in component "CT idler 3"
ref_plane "WorkPlane2" through (0, 0, 43.4) normal (0, 0, 1) x (1, 0, 0) in component "CT idler 3"
sketch "Sketch2 (3)" plane through (0, 0, 43.4) normal (0, 0, 1) x (1, 0, 0) in component "CT idler 3"
  line L0 (67.739, -50.3395) -> (68.0283, -50.385)
  line L1 (68.0283, -50.385) -> (68.1089, -50.3859)
  line L2 (68.1089, -50.3859) -> (68.1909, -50.3767)
  line L3 (68.1909, -50.3767) -> (68.2738, -50.3606)
  line L4 (68.2738, -50.3606) -> (68.3573, -50.3386)
  line L5 (68.3573, -50.3386) -> (68.4411, -50.3111)
  line L6 (68.4411, -50.3111) -> (68.5251, -50.2786)
  line L7 (68.5251, -50.2786) -> (68.6092, -50.2413)
  line L8 (68.6092, -50.2413) -> (68.6931, -50.1993)
  line L9 (68.6931, -50.1993) -> (68.7768, -50.1527)
  line L10 (68.7768, -50.1527) -> (68.86, -50.1017)
  line L11 (68.86, -50.1017) -> (68.9427, -50.0464)
  line L12 (68.9427, -50.0464) -> (69.0247, -49.9868)
  line L13 (69.0247, -49.9868) -> (69.0264, -49.9015)
  line L14 (69.0264, -49.9015) -> (69.0264, -49.8162)
  line L15 (69.0264, -49.8162) -> (69.0247, -49.7309)
  line L16 (69.0247, -49.7309) -> (68.9427, -49.6713)
  line L17 (68.9427, -49.6713) -> (68.86, -49.616)
  line L18 (68.86, -49.616) -> (68.7768, -49.565)
  line L19 (68.7768, -49.565) -> (68.6931, -49.5184)
  line L20 (68.6931, -49.5184) -> (68.6092, -49.4764)
  line L21 (68.6092, -49.4764) -> (68.5251, -49.439)
  line L22 (68.5251, -49.439) -> (68.4411, -49.4065)
  line L23 (68.4411, -49.4065) -> (68.3573, -49.3791)
  line L24 (68.3573, -49.3791) -> (68.2738, -49.357)
  line L25 (68.2738, -49.357) -> (68.1909, -49.3409)
  line L26 (68.1909, -49.3409) -> (68.1089, -49.3318)
  line L27 (68.1089, -49.3318) -> (68.0283, -49.3326)
  line L28 (68.0283, -49.3326) -> (67.739, -49.3782)
  line L29 (67.739, -49.3782) -> (67.7094, -49.2177)
  line L30 (67.7094, -49.2177) -> (67.6713, -49.0591)
  line L31 (67.6713, -49.0591) -> (67.6249, -48.9026)
  line L32 (67.6249, -48.9026) -> (67.5704, -48.7489)
  line L33 (67.5704, -48.7489) -> (67.8437, -48.6437)
  line L34 (67.8437, -48.6437) -> (67.9139, -48.6041)
  line L35 (67.9139, -48.6041) -> (67.9804, -48.5552)
  line L36 (67.9804, -48.5552) -> (68.0441, -48.4998)
  line L37 (68.0441, -48.4998) -> (68.1054, -48.439)
  line L38 (68.1054, -48.439) -> (68.1643, -48.3733)
  line L39 (68.1643, -48.3733) -> (68.2208, -48.3031)
  line L40 (68.2208, -48.3031) -> (68.2749, -48.2287)
  line L41 (68.2749, -48.2287) -> (68.3266, -48.1504)
  line L42 (68.3266, -48.1504) -> (68.3757, -48.0682)
  line L43 (68.3757, -48.0682) -> (68.4223, -47.9825)
  line L44 (68.4223, -47.9825) -> (68.4663, -47.8932)
  line L45 (68.4663, -47.8932) -> (68.5075, -47.8006)
  line L46 (68.5075, -47.8006) -> (68.4663, -47.7259)
  line L47 (68.4663, -47.7259) -> (68.4236, -47.652)
  line L48 (68.4236, -47.652) -> (68.3795, -47.579)
  line L49 (68.3795, -47.579) -> (68.2787, -47.5684)
  line L50 (68.2787, -47.5684) -> (68.1794, -47.5618)
  line L51 (68.1794, -47.5618) -> (68.0819, -47.5592)
  line L52 (68.0819, -47.5592) -> (67.9861, -47.5608)
  line L53 (67.9861, -47.5608) -> (67.8924, -47.5663)
  line L54 (67.8924, -47.5663) -> (67.801, -47.576)
  line L55 (67.801, -47.576) -> (67.712, -47.5898)
  line L56 (67.712, -47.5898) -> (67.6256, -47.608)
  line L57 (67.6256, -47.608) -> (67.5423, -47.6306)
  line L58 (67.5423, -47.6306) -> (67.4625, -47.6581)
  line L59 (67.4625, -47.6581) -> (67.3869, -47.6912)
  line L60 (67.3869, -47.6912) -> (67.3175, -47.7323)
  line L61 (67.3175, -47.7323) -> (67.0897, -47.9164)
  line L62 (67.0897, -47.9164) -> (66.9838, -47.7923)
  line L63 (66.9838, -47.7923) -> (66.8715, -47.6739)
  line L64 (66.8715, -47.6739) -> (66.7532, -47.5616)
  line L65 (66.7532, -47.5616) -> (66.629, -47.4557)
  line L66 (66.629, -47.4557) -> (66.8131, -47.2279)
  line L67 (66.8131, -47.2279) -> (66.8542, -47.1585)
  line L68 (66.8542, -47.1585) -> (66.8873, -47.0829)
  line L69 (66.8873, -47.0829) -> (66.9148, -47.0031)
  line L70 (66.9148, -47.0031) -> (66.9374, -46.9198)
  line L71 (66.9374, -46.9198) -> (66.9556, -46.8335)
  line L72 (66.9556, -46.8335) -> (66.9694, -46.7444)
  line L73 (66.9694, -46.7444) -> (66.9791, -46.653)
  line L74 (66.9791, -46.653) -> (66.9847, -46.5593)
  line L75 (66.9847, -46.5593) -> (66.9862, -46.4636)
  line L76 (66.9862, -46.4636) -> (66.9836, -46.366)
  line L77 (66.9836, -46.366) -> (66.9771, -46.2667)
  line L78 (66.9771, -46.2667) -> (66.9664, -46.1659)
  line L79 (66.9664, -46.1659) -> (66.8934, -46.1218)
  line L80 (66.8934, -46.1218) -> (66.8195, -46.0791)
  line L81 (66.8195, -46.0791) -> (66.7449, -46.0379)
  line L82 (66.7449, -46.0379) -> (66.6522, -46.0792)
  line L83 (66.6522, -46.0792) -> (66.563, -46.1231)
  line L84 (66.563, -46.1231) -> (66.4772, -46.1697)
  line L85 (66.4772, -46.1697) -> (66.395, -46.2189)
  line L86 (66.395, -46.2189) -> (66.3167, -46.2705)
  line L87 (66.3167, -46.2705) -> (66.2423, -46.3246)
  line L88 (66.2423, -46.3246) -> (66.1721, -46.3811)
  line L89 (66.1721, -46.3811) -> (66.1065, -46.44)
  line L90 (66.1065, -46.44) -> (66.0456, -46.5013)
  line L91 (66.0456, -46.5013) -> (65.9903, -46.565)
  line L92 (65.9903, -46.565) -> (65.9413, -46.6315)
  line L93 (65.9413, -46.6315) -> (65.9017, -46.7017)
  line L94 (65.9017, -46.7017) -> (65.7965, -46.9751)
  line L95 (65.7965, -46.9751) -> (65.6428, -46.9205)
  line L96 (65.6428, -46.9205) -> (65.4863, -46.8741)
  line L97 (65.4863, -46.8741) -> (65.3277, -46.8361)
  line L98 (65.3277, -46.8361) -> (65.1672, -46.8064)
  line L99 (65.1672, -46.8064) -> (65.2128, -46.5171)
  line L100 (65.2128, -46.5171) -> (65.2136, -46.4365)
  line L101 (65.2136, -46.4365) -> (65.2045, -46.3545)
  line L102 (65.2045, -46.3545) -> (65.1884, -46.2716)
  line L103 (65.1884, -46.2716) -> (65.1663, -46.1881)
  line L104 (65.1663, -46.1881) -> (65.1389, -46.1043)
  line L105 (65.1389, -46.1043) -> (65.1064, -46.0203)
  line L106 (65.1064, -46.0203) -> (65.069, -45.9362)
  line L107 (65.069, -45.9362) -> (65.027, -45.8523)
  line L108 (65.027, -45.8523) -> (64.9805, -45.7687)
  line L109 (64.9805, -45.7687) -> (64.9295, -45.6854)
  line L110 (64.9295, -45.6854) -> (64.8741, -45.6027)
  line L111 (64.8741, -45.6027) -> (64.8145, -45.5207)
  line L112 (64.8145, -45.5207) -> (64.7292, -45.519)
  line L113 (64.7292, -45.519) -> (64.6439, -45.519)
  line L114 (64.6439, -45.519) -> (64.5587, -45.5207)
  line L115 (64.5587, -45.5207) -> (64.499, -45.6027)
  line L116 (64.499, -45.6027) -> (64.4437, -45.6854)
  line L117 (64.4437, -45.6854) -> (64.3927, -45.7687)
  line L118 (64.3927, -45.7687) -> (64.3462, -45.8523)
  line L119 (64.3462, -45.8523) -> (64.3041, -45.9362)
  line L120 (64.3041, -45.9362) -> (64.2668, -46.0203)
  line L121 (64.2668, -46.0203) -> (64.2343, -46.1043)
  line L122 (64.2343, -46.1043) -> (64.2068, -46.1881)
  line L123 (64.2068, -46.1881) -> (64.1848, -46.2716)
  line L124 (64.1848, -46.2716) -> (64.1687, -46.3545)
  line L125 (64.1687, -46.3545) -> (64.1595, -46.4365)
  line L126 (64.1595, -46.4365) -> (64.1604, -46.5171)
  line L127 (64.1604, -46.5171) -> (64.206, -46.8064)
  line L128 (64.206, -46.8064) -> (64.0455, -46.8361)
  line L129 (64.0455, -46.8361) -> (63.8868, -46.8741)
  line L130 (63.8868, -46.8741) -> (63.7304, -46.9205)
  line L131 (63.7304, -46.9205) -> (63.5766, -46.9751)
  line L132 (63.5766, -46.9751) -> (63.4714, -46.7017)
  line L133 (63.4714, -46.7017) -> (63.4319, -46.6315)
  line L134 (63.4319, -46.6315) -> (63.3829, -46.565)
  line L135 (63.3829, -46.565) -> (63.3275, -46.5013)
  line L136 (63.3275, -46.5013) -> (63.2667, -46.44)
  line L137 (63.2667, -46.44) -> (63.201, -46.3811)
  line L138 (63.201, -46.3811) -> (63.1309, -46.3246)
  line L139 (63.1309, -46.3246) -> (63.0565, -46.2705)
  line L140 (63.0565, -46.2705) -> (62.9781, -46.2189)
  line L141 (62.9781, -46.2189) -> (62.896, -46.1697)
  line L142 (62.896, -46.1697) -> (62.8102, -46.1231)
  line L143 (62.8102, -46.1231) -> (62.7209, -46.0792)
  line L144 (62.7209, -46.0792) -> (62.6283, -46.0379)
  line L145 (62.6283, -46.0379) -> (62.5536, -46.0791)
  line L146 (62.5536, -46.0791) -> (62.4798, -46.1218)
  line L147 (62.4798, -46.1218) -> (62.4067, -46.1659)
  line L148 (62.4067, -46.1659) -> (62.3961, -46.2667)
  line L149 (62.3961, -46.2667) -> (62.3895, -46.366)
  line L150 (62.3895, -46.366) -> (62.387, -46.4636)
  line L151 (62.387, -46.4636) -> (62.3885, -46.5593)
  line L152 (62.3885, -46.5593) -> (62.3941, -46.653)
  line L153 (62.3941, -46.653) -> (62.4038, -46.7444)
  line L154 (62.4038, -46.7444) -> (62.4176, -46.8335)
  line L155 (62.4176, -46.8335) -> (62.4357, -46.9198)
  line L156 (62.4357, -46.9198) -> (62.4584, -47.0031)
  line L157 (62.4584, -47.0031) -> (62.4859, -47.0829)
  line L158 (62.4859, -47.0829) -> (62.519, -47.1585)
  line L159 (62.519, -47.1585) -> (62.56, -47.2279)
  line L160 (62.56, -47.2279) -> (62.7441, -47.4557)
  line L161 (62.7441, -47.4557) -> (62.62, -47.5616)
  line L162 (62.62, -47.5616) -> (62.5016, -47.6739)
  line L163 (62.5016, -47.6739) -> (62.3893, -47.7923)
  line L164 (62.3893, -47.7923) -> (62.2835, -47.9164)
  line L165 (62.2835, -47.9164) -> (62.0557, -47.7323)
  line L166 (62.0557, -47.7323) -> (61.9863, -47.6912)
  line L167 (61.9863, -47.6912) -> (61.9107, -47.6581)
  line L168 (61.9107, -47.6581) -> (61.8308, -47.6306)
  line L169 (61.8308, -47.6306) -> (61.7475, -47.608)
  line L170 (61.7475, -47.608) -> (61.6612, -47.5898)
  line L171 (61.6612, -47.5898) -> (61.5722, -47.576)
  line L172 (61.5722, -47.576) -> (61.4807, -47.5663)
  line L173 (61.4807, -47.5663) -> (61.387, -47.5608)
  line L174 (61.387, -47.5608) -> (61.2913, -47.5592)
  line L175 (61.2913, -47.5592) -> (61.1937, -47.5618)
  line L176 (61.1937, -47.5618) -> (61.0945, -47.5684)
  line L177 (61.0945, -47.5684) -> (60.9936, -47.579)
  line L178 (60.9936, -47.579) -> (60.9495, -47.652)
  line L179 (60.9495, -47.652) -> (60.9069, -47.7259)
  line L180 (60.9069, -47.7259) -> (60.8657, -47.8006)
  line L181 (60.8657, -47.8006) -> (60.9069, -47.8932)
  line L182 (60.9069, -47.8932) -> (60.9509, -47.9825)
  line L183 (60.9509, -47.9825) -> (60.9975, -48.0682)
  line L184 (60.9975, -48.0682) -> (61.0466, -48.1504)
  line L185 (61.0466, -48.1504) -> (61.0983, -48.2287)
  line L186 (61.0983, -48.2287) -> (61.1524, -48.3031)
  line L187 (61.1524, -48.3031) -> (61.2089, -48.3733)
  line L188 (61.2089, -48.3733) -> (61.2678, -48.439)
  line L189 (61.2678, -48.439) -> (61.329, -48.4998)
  line L190 (61.329, -48.4998) -> (61.3928, -48.5552)
  line L191 (61.3928, -48.5552) -> (61.4593, -48.6041)
  line L192 (61.4593, -48.6041) -> (61.5295, -48.6437)
  line L193 (61.5295, -48.6437) -> (61.8028, -48.7489)
  line L194 (61.8028, -48.7489) -> (61.7483, -48.9026)
  line L195 (61.7483, -48.9026) -> (61.7019, -49.0591)
  line L196 (61.7019, -49.0591) -> (61.6638, -49.2177)
  line L197 (61.6638, -49.2177) -> (61.6342, -49.3782)
  line L198 (61.6342, -49.3782) -> (61.3449, -49.3326)
  line L199 (61.3449, -49.3326) -> (61.2643, -49.3318)
  line L200 (61.2643, -49.3318) -> (61.1822, -49.3409)
  line L201 (61.1822, -49.3409) -> (61.0993, -49.357)
  line L202 (61.0993, -49.357) -> (61.0159, -49.3791)
  line L203 (61.0159, -49.3791) -> (60.932, -49.4065)
  line L204 (60.932, -49.4065) -> (60.848, -49.439)
  line L205 (60.848, -49.439) -> (60.764, -49.4764)
  line L206 (60.764, -49.4764) -> (60.6801, -49.5184)
  line L207 (60.6801, -49.5184) -> (60.5964, -49.565)
  line L208 (60.5964, -49.565) -> (60.5132, -49.616)
  line L209 (60.5132, -49.616) -> (60.4305, -49.6713)
  line L210 (60.4305, -49.6713) -> (60.3485, -49.7309)
  line L211 (60.3485, -49.7309) -> (60.3468, -49.8162)
  line L212 (60.3468, -49.8162) -> (60.3468, -49.9015)
  line L213 (60.3468, -49.9015) -> (60.3485, -49.9868)
  line L214 (60.3485, -49.9868) -> (60.4305, -50.0464)
  line L215 (60.4305, -50.0464) -> (60.5132, -50.1017)
  line L216 (60.5132, -50.1017) -> (60.5964, -50.1527)
  line L217 (60.5964, -50.1527) -> (60.6801, -50.1993)
  line L218 (60.6801, -50.1993) -> (60.764, -50.2413)
  line L219 (60.764, -50.2413) -> (60.848, -50.2786)
  line L220 (60.848, -50.2786) -> (60.932, -50.3111)
  line L221 (60.932, -50.3111) -> (61.0159, -50.3386)
  line L222 (61.0159, -50.3386) -> (61.0993, -50.3606)
  line L223 (61.0993, -50.3606) -> (61.1822, -50.3767)
  line L224 (61.1822, -50.3767) -> (61.2643, -50.3859)
  line L225 (61.2643, -50.3859) -> (61.3449, -50.385)
  line L226 (61.3449, -50.385) -> (61.6342, -50.3395)
  line L227 (61.6342, -50.3395) -> (61.6638, -50.4999)
  line L228 (61.6638, -50.4999) -> (61.7019, -50.6586)
  line L229 (61.7019, -50.6586) -> (61.7483, -50.815)
  line L230 (61.7483, -50.815) -> (61.8028, -50.9688)
  line L231 (61.8028, -50.9688) -> (61.5295, -51.074)
  line L232 (61.5295, -51.074) -> (61.4593, -51.1135)
  line L233 (61.4593, -51.1135) -> (61.3928, -51.1625)
  line L234 (61.3928, -51.1625) -> (61.329, -51.2179)
  line L235 (61.329, -51.2179) -> (61.2678, -51.2787)
  line L236 (61.2678, -51.2787) -> (61.2089, -51.3444)
  line L237 (61.2089, -51.3444) -> (61.1524, -51.4146)
  line L238 (61.1524, -51.4146) -> (61.0983, -51.4889)
  line L239 (61.0983, -51.4889) -> (61.0466, -51.5673)
  line L240 (61.0466, -51.5673) -> (60.9975, -51.6494)
  line L241 (60.9975, -51.6494) -> (60.9509, -51.7352)
  line L242 (60.9509, -51.7352) -> (60.9069, -51.8245)
  line L243 (60.9069, -51.8245) -> (60.8657, -51.9171)
  line L244 (60.8657, -51.9171) -> (60.9069, -51.9918)
  line L245 (60.9069, -51.9918) -> (60.9495, -52.0657)
  line L246 (60.9495, -52.0657) -> (60.9936, -52.1387)
  line L247 (60.9936, -52.1387) -> (61.0945, -52.1493)
  line L248 (61.0945, -52.1493) -> (61.1937, -52.1559)
  line L249 (61.1937, -52.1559) -> (61.2913, -52.1584)
  line L250 (61.2913, -52.1584) -> (61.387, -52.1569)
  line L251 (61.387, -52.1569) -> (61.4807, -52.1513)
  line L252 (61.4807, -52.1513) -> (61.5722, -52.1417)
  line L253 (61.5722, -52.1417) -> (61.6612, -52.1278)
  line L254 (61.6612, -52.1278) -> (61.7475, -52.1097)
  line L255 (61.7475, -52.1097) -> (61.8308, -52.087)
  line L256 (61.8308, -52.087) -> (61.9107, -52.0595)
  line L257 (61.9107, -52.0595) -> (61.9863, -52.0264)
  line L258 (61.9863, -52.0264) -> (62.0557, -51.9854)
  line L259 (62.0557, -51.9854) -> (62.2835, -51.8013)
  line L260 (62.2835, -51.8013) -> (62.3893, -51.9254)
  line L261 (62.3893, -51.9254) -> (62.5016, -52.0438)
  line L262 (62.5016, -52.0438) -> (62.62, -52.1561)
  line L263 (62.62, -52.1561) -> (62.7441, -52.262)
  line L264 (62.7441, -52.262) -> (62.56, -52.4897)
  line L265 (62.56, -52.4897) -> (62.519, -52.5591)
  line L266 (62.519, -52.5591) -> (62.4859, -52.6347)
  line L267 (62.4859, -52.6347) -> (62.4584, -52.7146)
  line L268 (62.4584, -52.7146) -> (62.4357, -52.7979)
  line L269 (62.4357, -52.7979) -> (62.4176, -52.8842)
  line L270 (62.4176, -52.8842) -> (62.4038, -52.9732)
  line L271 (62.4038, -52.9732) -> (62.3941, -53.0647)
  line L272 (62.3941, -53.0647) -> (62.3885, -53.1584)
  line L273 (62.3885, -53.1584) -> (62.387, -53.2541)
  line L274 (62.387, -53.2541) -> (62.3895, -53.3517)
  line L275 (62.3895, -53.3517) -> (62.3961, -53.451)
  line L276 (62.3961, -53.451) -> (62.4067, -53.5518)
  line L277 (62.4067, -53.5518) -> (62.4798, -53.5959)
  line L278 (62.4798, -53.5959) -> (62.5536, -53.6385)
  line L279 (62.5536, -53.6385) -> (62.6283, -53.6797)
  line L280 (62.6283, -53.6797) -> (62.7209, -53.6385)
  line L281 (62.7209, -53.6385) -> (62.8102, -53.5946)
  line L282 (62.8102, -53.5946) -> (62.896, -53.548)
  line L283 (62.896, -53.548) -> (62.9781, -53.4988)
  line L284 (62.9781, -53.4988) -> (63.0565, -53.4471)
  line L285 (63.0565, -53.4471) -> (63.1309, -53.393)
  line L286 (63.1309, -53.393) -> (63.201, -53.3365)
  line L287 (63.201, -53.3365) -> (63.2667, -53.2776)
  line L288 (63.2667, -53.2776) -> (63.3275, -53.2164)
  line L289 (63.3275, -53.2164) -> (63.3829, -53.1526)
  line L290 (63.3829, -53.1526) -> (63.4319, -53.0862)
  line L291 (63.4319, -53.0862) -> (63.4714, -53.0159)
  line L292 (63.4714, -53.0159) -> (63.5766, -52.7426)
  line L293 (63.5766, -52.7426) -> (63.7304, -52.7972)
  line L294 (63.7304, -52.7972) -> (63.8868, -52.8435)
  line L295 (63.8868, -52.8435) -> (64.0455, -52.8816)
  line L296 (64.0455, -52.8816) -> (64.206, -52.9112)
  line L297 (64.206, -52.9112) -> (64.1604, -53.2005)
  line L298 (64.1604, -53.2005) -> (64.1595, -53.2811)
  line L299 (64.1595, -53.2811) -> (64.1687, -53.3632)
  line L300 (64.1687, -53.3632) -> (64.1848, -53.4461)
  line L301 (64.1848, -53.4461) -> (64.2068, -53.5295)
  line L302 (64.2068, -53.5295) -> (64.2343, -53.6134)
  line L303 (64.2343, -53.6134) -> (64.2668, -53.6974)
  line L304 (64.2668, -53.6974) -> (64.3041, -53.7814)
  line L305 (64.3041, -53.7814) -> (64.3462, -53.8654)
  line L306 (64.3462, -53.8654) -> (64.3927, -53.949)
  line L307 (64.3927, -53.949) -> (64.4437, -54.0323)